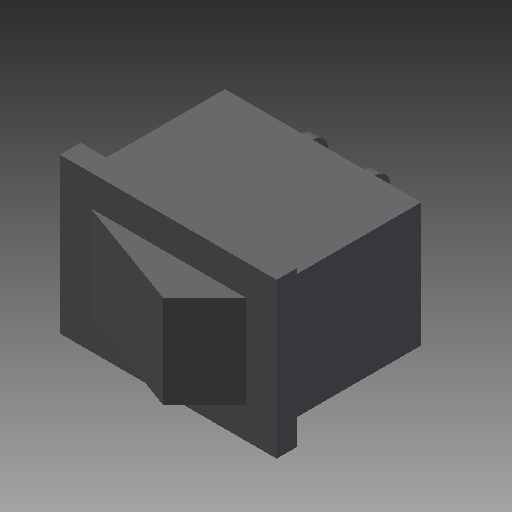
# Autodesk Inventor part: sw
Saved by Autodesk Inventor 2018 (Build 220112000, 112)
## iProperties
Category: コックピット
Shininess: 64.0
Length Units: 11269
Angle Units: 11279
Time Units: 11290
Mass Units: 11284
Length Display Precision: 3
Angle Display Precision: 2
Compacted: True
Part Number: sw
Document SubType Name: Modeling
Created: 2003-12-02
Designer: hajime
Manufacturer: Standard
Standards Organization: Custom
Material: ABS Plastic
Density: 1.06 g/cm^3
Appearance: Grey (Dark)
Density: 0.0
Volumn: 0.0
Area: 0.0
PropertySet Name: Model Information
Control State: 0
Master: False
Checked Out: False
Author: hajime
Autodesk Inventor part; units mm, degrees
ref_plane "YZ Plane" through (0, 0, 0) normal (1, 0, 0) x (0, 1, 0)
ref_plane "XZ Plane" through (0, 0, 0) normal (0, 1, 0) x (-1, 0, 0)
ref_plane "XY Plane" through (0, 0, 0) normal (0, 0, 1) x (1, 0, 0)
sketch "スケッチ1" plane through (0, 0, 0) normal (0, 0, 1) x (1, 0, 0)
  line L0 (-9.1992, 6.0057) -> (9.8008, 6.0057)
  line L1 (9.8008, 6.0057) -> (9.8008, -5.9943)
  line L2 (9.8008, -5.9943) -> (-9.1992, -5.9943)
  line L3 (-9.1992, -5.9943) -> (-9.1992, 6.0057)
  dimension "d0" = 19
  dimension "d1" = 12
  constraints: 8 end point, 2 parallel, 1 horizontal, 1 perpendicular
  measures "d0" distance of L0.start L0.end
  measures "d1" distance of L0.end L1.end
extrude "押し出し1" add sketch "スケッチ1" along normal blind 13
sketch "スケッチ2" plane through (0, 0, 13) normal (0, 0, 1) x (1, 0, 0)
  line L0 (-9.1992, 6.0057) -> (9.8008, 6.0057) projected
  line L1 (-9.1992, -5.9943) -> (-9.1992, 6.0057) projected
  line L2 (-10.1992, 7.5057) -> (10.8008, 7.5057)
  line L3 (10.8008, 7.5057) -> (10.8008, -7.4943)
  line L4 (10.8008, -7.4943) -> (-10.1992, -7.4943)
  line L5 (-10.1992, -7.4943) -> (-10.1992, 7.5057)
  dimension "d4" = 21
  dimension "d5" = 15
  dimension "d6" = 1.5
  dimension "d7" = 1
  constraints: 8 end point, 2 parallel, 1 horizontal, 1 perpendicular
  measures "d4" distance of L2.start L2.end
  measures "d5" distance of L4.end L2.start
  measures "d6" distance between parallel lines of L0 L2
  measures "d7" distance between parallel lines of L5 L1
extrude "押し出し2" add sketch "スケッチ2" along normal blind 2
sketch "スケッチ3" plane through (0, 0, 15) normal (0, 0, 1) x (1, 0, 0)
  line L0 (-10.1992, 7.5057) -> (10.8008, 7.5057) projected
  line L1 (-10.1992, -7.4943) -> (-10.1992, 7.5057) projected
  line L2 (-7.1992, 4.5057) -> (7.8008, 4.5057)
  line L3 (7.8008, 4.5057) -> (7.8008, -4.4943)
  line L4 (7.8008, -4.4943) -> (-7.1992, -4.4943)
  line L5 (-7.1992, -4.4943) -> (-7.1992, 4.5057)
  dimension "d10" = 9
  dimension "d11" = 15
  dimension "d12" = 3
  dimension "d13" = 3
  constraints: 8 end point, 2 parallel, 1 horizontal, 1 perpendicular
  measures "d10" distance of L4.end L2.start
  measures "d11" distance of L2.start L2.end
  measures "d12" distance between parallel lines of L0 L2
  measures "d13" distance between parallel lines of L1 L5
extrude "押し出し3" add sketch "スケッチ3" along normal blind 4
chamfer "面取り1" distance 4 distance2 11 1 edges at (-7.1992, 0.0057, 19) measured on face at (-7.1992, -1.4943, 16.3333)
chamfer "面取り2" distance 4 distance2 4 1 edges at (7.8008, 0.0057, 19) measured on face at (7.8008, 1.5057, 16.3333)
sketch "スケッチ4" plane through (0, 0, 0) normal (0, 0, -1) x (-1, 0, 0)
  line L0 (9.1992, 6.0057) -> (-9.8008, 6.0057) projected
  line L1 (9.1992, -5.9943) -> (9.1992, 6.0057) projected
  line L2 (-0.8008, 1.5057) -> (0.1992, 1.5057)
  line L3 (0.1992, 1.5057) -> (0.1992, -1.4943)
  line L4 (0.1992, -1.4943) -> (-0.8008, -1.4943)
  line L5 (-0.8008, -1.4943) -> (-0.8008, 1.5057)
  line L6 (5.1992, 1.5057) -> (6.1992, 1.5057)
  line L7 (6.1992, 1.5057) -> (6.1992, -1.4943)
  line L8 (6.1992, -1.4943) -> (5.1992, -1.4943)
  line L9 (5.1992, -1.4943) -> (5.1992, 1.5057)
  dimension "d20" = 9
  dimension "d21" = 1
  dimension "d22" = 3
  dimension "d23" = 4.5
  dimension "d24" = 1
  dimension "d25" = 5
  constraints: 16 end point, 4 parallel, 2 collinear, 2 horizontal, 2 perpendicular
  measures "d20" distance between parallel lines of L3 L1
  measures "d21" distance of L2.start L2.end
  measures "d22" distance of L4.end L2.start
  measures "d23" distance between parallel lines of L0 L2
  measures "d24" distance of L6.start L6.end
  measures "d25" distance between parallel lines of L3 L9
extrude "押し出し4" add sketch "スケッチ4" along normal blind 6
fillet "フィレット1" radius 1.5 4 edges at (0.3008, 1.5057, -6) (0.3008, -1.4943, -6) (-5.6992, -1.4943, -6) (-5.6992, 1.5057, -6)
